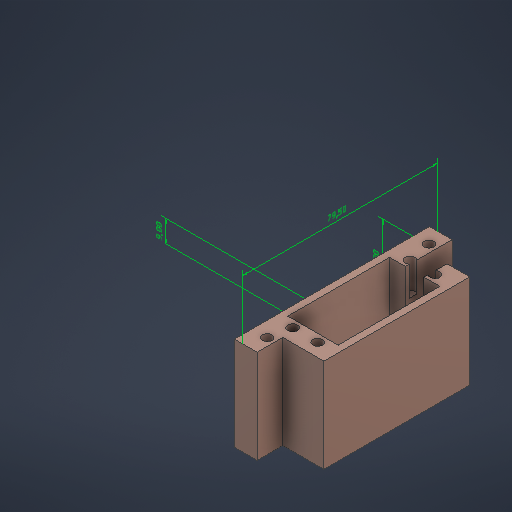
# Autodesk Inventor part: Case servo MG
Saved by Autodesk Inventor 2026 (Build 300175000, 175)
## iProperties
Created: 2025-08-24
Part Number: Case servo MG
Material: Plástico PC/ABS
Document SubType Name: Modeling
Designer: Thomas
Density: 1.1 g/cm^3
Appearance: Suave - Blanco
Author: Thomas
Autodesk Inventor part; units mm, degrees
ref_plane "YZ Plane" through (0, 0, 0) normal (1, 0, 0) x (0, 1, 0)
ref_plane "XZ Plane" through (0, 0, 0) normal (0, 1, 0) x (-1, 0, 0)
ref_plane "XY Plane" through (0, 0, 0) normal (0, 0, 1) x (1, 0, 0)
sketch "Boceto1" plane through (0, 0, 0) normal (1, 0, 0) x (0, 1, 0)
  line L0 (36.2, -20.75) -> (9, -20.75)
  line L1 (9, -20.75) -> (9, 20.75)
  line L2 (9, 20.75) -> (36.2, 20.75)
  line L3 (36.2, 20.75) -> (36.2, -20.75)
  line L4 (36.2, -29.75) -> (0, -29.75)
  line L5 (0, -29.75) -> (0, 29.75)
  line L6 (0, 29.75) -> (36.2, 29.75)
  line L7 (36.2, -29.75) -> (36.2, -20.75)
  line L8 (36.2, 20.75) -> (36.2, 29.75)
  point P0 (0, 0)
  point P1 (0, 0)
  dimension "d0" = 41.5
  dimension "d1" = 27.2
  dimension "d4" = 9
  constraints: 18 end point, 4 equal length, 2 perpendicular, 2 vertical alignment, 1 coincident, 1 horizontal, 1 midpoint, 1 vertical, 2 other
  measures "d0" distance of L0.end L1.end
  measures "d1" distance of L0.start L0.end
  measures "d4" distance between parallel lines of L1 L5
extrude "Extrusión1" add sketch "Boceto1" along normal mid plane 26
extrude "Extrusión2" cut sketch "Boceto1" along normal mid plane 20.5 contours L0 L1 L2 L3
sketch "Boceto2" plane through (-13, 0, 29.75) normal (0, 0, 1) x (1, 0, 0)
  line L0 (23.25, 36.2) -> (2.75, 36.2) projected
  line L1 (9.25, 36.2) -> (16.75, 36.2)
  line L2 (16.75, 36.2) -> (16.75, 8.2)
  line L3 (16.75, 8.2) -> (9.25, 8.2)
  line L4 (9.25, 8.2) -> (9.25, 36.2)
  line L5 (0, 0) -> (26, 0) projected
  point P0 (13, 0)
  point P1 (13, 36.2)
  dimension "d9" = 7.5
  dimension "d10" = 8.2
  constraints: 8 end point, 2 midpoint, 2 parallel, 1 horizontal, 1 perpendicular, 1 point on line
  measures "d9" distance of L2.end L3.end
  measures "d10" distance between parallel lines of L3 L5
extrude "Extrusión3" cut sketch "Boceto2" against normal up to surface (9 mm away) from surface at -50.5
sketch "Boceto3" plane through (0, 0, 0) normal (1, 0, 0) x (0, 1, 0)
  line L0 (9, -20.75) -> (9, 20.75) projected
  line L1 (0, 29.75) -> (0, -29.75) projected
  line L2 (9, 0) -> (0, 0)
  line L3 (0, 0) -> (0, -1.75)
  line L4 (0, -1.75) -> (9, -1.75)
  line L5 (9, -1.75) -> (9, 0)
  line L6 (0, -29.75) -> (0, 29.75) projected
  line L7 (9, 0) -> (2, 0)
  line L8 (2, 0) -> (2, -3.4)
  line L9 (2, -3.4) -> (9, -3.4)
  line L10 (9, -3.4) -> (9, 0)
  point P0 (0, 0)
  point P1 (0, 0)
  point P2 (9, -1.75)
  point P3 (0, 0)
  point P4 (5.5, 0)
  point P5 (9, -3.4)
  point P6 (2, -1.75)
  dimension "d13" = 1.75
  dimension "d15" = 3.4
  dimension "d16" = 2
  constraints: 16 end point, 4 parallel, 3 midpoint, 2 horizontal, 2 perpendicular, 1 point on line
  measures "d13" distance from line of point (0, 0) L4
  measures "d15" distance from line of point (5.5, 0) L9
  measures "d16" distance between parallel lines of L8 L1
revolve "Revolución1" cut sketch "Boceto3" angle 360 about axis through (0, 9, 0) along (0, -1, 0)
sketch "Boceto4" plane through (-13, 36.2, 29.75) normal (0, 1, 0) x (1, 0, 0)
  arc A0 (19.25, 3.9745) -> (16.95, 3.9745) centre (18.1, 5.85) ccw projected
  arc A1 (9.05, 3.9745) -> (6.75, 3.9745) centre (7.9, 5.85) ccw projected
  arc A2 (16.95, 55.5255) -> (19.25, 55.5255) centre (18.1, 53.65) ccw projected
  arc A3 (6.75, 55.5255) -> (9.05, 55.5255) centre (7.9, 53.65) ccw projected
  circle A4 centre (18.1, 53.65) radius 2
  circle A5 centre (7.9, 53.65) radius 2
  circle A6 centre (18.1, 5.85) radius 2
  circle A7 centre (7.9, 5.85) radius 2
  point P0 (13, 29.75)
  dimension "d17" = 4
  dimension "d18" = 4
  dimension "d19" = 4
  dimension "d20" = 4
  constraints: 4 centre point, 4 coincident
  measures "d17" diameter of A4
  measures "d18" diameter of A5
  measures "d19" diameter of A6
  measures "d20" diameter of A7
extrude "Extrusión4" cut sketch "Boceto4" against normal blind 10
sketch "Boceto5" plane through (13, 0, -29.75) normal (0, 0, -1) x (-1, 0, 0)
  line L0 (16.75, 36.2) -> (16.75, 8.2) projected
  line L1 (16.75, 36.2) -> (26, 36.2)
  line L2 (26, 36.2) -> (26, 0)
  line L3 (26, 0) -> (16.75, 0)
  line L4 (16.75, 0) -> (16.75, 36.2)
  point P0 (13, 0)
  point P1 (16.75, 8.2)
  constraints: 8 end point, 2 parallel, 1 horizontal, 1 perpendicular
extrude "Extrusión5" add sketch "Boceto5" along normal blind 10
mirror "Simetría1" about plane through (0, 0, 0) normal (0, 0, 1) of "Extrusión5"
sketch "Boceto6" plane through (13, 0, -29.75) normal (0, -1, 0) x (1, 0, 0)
  circle A0 centre (-13.2277, 36.7463) radius 0.75 projected
  circle A1 centre (-6.0037, 29.9777) radius 0.75 projected
  line L0 (-4, 19.95) -> (-22, 19.95) projected
  circle A2 centre (-12.7723, 22.7537) radius 0.75 projected
  circle A3 centre (-19.9963, 29.5223) radius 0.75 projected
  point P0 (-13, 29.75)
extrude "Extrusión6" cut sketch "Boceto6" against normal blind 8
sketch "Boceto7" plane through (13, 0, -29.75) normal (0, 0, -1) x (-1, 0, 0)
  line L0 (16.75, 0) -> (16.75, 8.2) projected
  line L1 (16.75, 8.2) -> (9.25, 8.2) projected
  line L2 (9.25, 8.2) -> (9.25, 36.2) projected
  line L3 (0, 36.2) -> (9.25, 36.2) projected
  line L4 (0, 0) -> (0, 36.2) projected
  line L5 (16.75, 0) -> (0, 0) projected
  point P0 (13, 0)
extrude "Extrusión7" add sketch "Boceto7" along normal blind 0.45
sketch "Boceto8" plane through (13, 0, 29.75) normal (0, 0, 1) x (1, 0, 0)
  line L0 (-16.75, 36.2) -> (-16.75, 0) projected
  line L1 (-16.75, 0) -> (0, 0) projected
  line L2 (0, 36.2) -> (0, 0) projected
  line L3 (-16.75, 36.2) -> (0, 36.2) projected
  point P0 (-13, 0)
extrude "Extrusión8" cut sketch "Boceto8" against normal blind 0.45
sketch "Boceto9" plane through (-10.25, 36.2, 20.75) normal (0, 1, 0) x (1, 0, 0)
  circle A0 centre (3.375, 54.225) radius 1.75 projected
  circle A1 centre (3.375, -11.825) radius 1.78 projected
  circle A2 centre (3.375, 54.225) radius 2
  circle A3 centre (3.375, -11.825) radius 2
  point P0 (10.25, 20.75)
  dimension "d43" = 4
  dimension "d44" = 4
  constraints: 2 centre point, 2 coincident
  measures "d43" diameter of A2
  measures "d44" diameter of A3
extrude "Extrusión9" cut sketch "Boceto9" against normal blind 5 contours A0 | A1 | A2 | A3
sketch "Boceto10" plane through (-13, 0, 0) normal (-1, 0, 0) x (0, 0, 1)
  circle A0 centre (28.75, 25.2) radius 1.75 projected
  circle A1 centre (-34.75, 25.2) radius 1.75 projected
  circle A2 centre (-34.75, 25.2) radius 2
  circle A3 centre (28.75, 25.2) radius 2
  point P0 (0, 0)
  dimension "d47" = 4
  dimension "d48" = 4
  constraints: 2 centre point, 2 coincident
  measures "d47" diameter of A2
  measures "d48" diameter of A3
extrude "Extrusión10" cut sketch "Boceto10" against normal blind 7 contours A0 | A1 | A2 | A3
move faces "Desplazar1" translate (0, 2, 0) faces at (-12.0833, 36.2, -6.9167)
equation "\"d18\" = d17"
equation "\"d19\" = d17"
equation "\"d20\" = d17"
equation "\"d43\" = d44"
equation "\"d48\" = d47"
